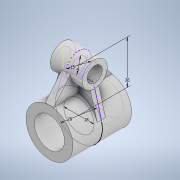
# Autodesk Inventor part: Part1
Saved by Autodesk Inventor 2022 (Build 260153000, 153)
## iProperties
Created: 2022-03-21
Part Number: Part1
Material: Generic
Document SubType Name: Modeling
Designer: HP RADEON
Density: 1 g/cm^3
Appearance: Default
Author: HP RADEON
Autodesk Inventor part; units mm, degrees
ref_plane "YZ Plane" through (0, 0, 0) normal (1, 0, 0) x (0, 1, 0)
ref_plane "XZ Plane" through (0, 0, 0) normal (0, 1, 0) x (-1, 0, 0)
ref_plane "XY Plane" through (0, 0, 0) normal (0, 0, 1) x (1, 0, 0)
sketch "Sketch1" plane through (0, 0, 0) normal (0, 0, 1) x (1, 0, 0)
  circle A0 centre (0, 0) radius 14
  circle A1 centre (0, 0) radius 9
  dimension "d0" = 28
  dimension "d1" = 18
  constraints: 2 centre point, 2 coincident
  measures "d0" diameter of A0
  measures "d1" diameter of A1
sketch "Sketch2" plane through (0, 0, 0) normal (1, 0, 0) x (0, 1, 0)
  circle A0 centre (26, 0) radius 7.5
  circle A1 centre (26, 0) radius 4.5
  point P0 (0, 0)
  dimension "d2" = 15
  dimension "d3" = 9
  dimension "d4" = 26
  constraints: 2 centre point, 1 coincident
  measures "d2" diameter of A0
  measures "d3" diameter of A1
  measures "d4" distance of point (0, 0) A0.centre
extrude "Extrusion1" add sketch "Sketch2" along normal mid plane 19
extrude "Extrusion2" add sketch "Sketch1" along normal mid plane 35
sketch "Sketch8" plane through (0, 0, 0) normal (1, 0, 0) x (0, 1, 0)
  circle A0 centre (26, 0) radius 7.5 projected
  line L0 (26, -7.5) -> (14, -17.4622)
  line L1 (14, 17.5) -> (-14, 17.5) projected
  line L2 (14, -17.4622) -> (14, 17.5)
  line L3 (14, 17.5) -> (26, 7.5)
  point P0 (0, 0)
  constraints: 6 end point, 2 point on circle
extrude "Extrusion5" add sketch "Sketch8" along normal mid plane 5 contours A0 L0 L2 L3
sketch "Sketch9" plane through (0, 0, 0) normal (1, 0, 0) x (0, 1, 0)
  circle A0 centre (26, 0) radius 7.5 projected
  point P0 (0, 0)
sketch "Sketch10" plane through (9.5, 26, 0) normal (1, 0, 0) x (0, 0, -1)
  point P0 (0, -26)
sketch "Sketch11" plane through (0, 0, 0) normal (0, 0, 1) x (1, 0, 0)
  line L0 (-9.5, 33.5) -> (-9.5, 18.5) projected
  line L1 (-9.5, 18.5) -> (-13.5146, 3.6547)
  circle A0 centre (0, 0) radius 14 projected
  line L2 (-9.5, 18.5) -> (9.5, 18.5) projected
  line L3 (8.6724, 21.4861) -> (13.4458, 4.3294)
  arc A1 (13.3262, 4.2909) -> (-13.5146, 3.6547) centre (0, 0) ccw
  arc A2 (13.3262, 4.2909) -> (0.3318, 13.9961) centre (0, 0) ccw
  arc A3 (13.4458, 4.3294) -> (-13.022, 5.476) centre (0, 0.0121) ccw
  line L4 (8.6724, 21.4861) -> (-8.6887, 21.5)
  line L5 (9.5, 21.5) -> (-9.5, 21.5) projected
  line L6 (-9.5, 18.5) -> (-8.6887, 21.5)
  point P0 (-13.022, 5.476)
  point P1 (13.4458, 4.3294)
  constraints: 8 end point, 7 point on circle, 3 centre point, 2 coincident, 2 point on line, 3 other
extrude "Extrusion6" add sketch "Sketch11" along normal mid plane 5 contours L6 L4 L3 A3 L1
sketch "Sketch12" plane through (13.4458, 4.3294, 2.5) normal (0.9634071, 0.2680423, 0) x (0, 0, -1)
  point P0 (2.5, -0.5669)
body "Solid1"
